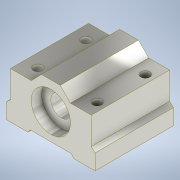
# Autodesk Inventor part: Balero lineal
Saved by Autodesk Inventor 2022 (Build 260153000, 153)
## iProperties
Created: 2021-11-08
Part Number: Balero lineal
Material: Steel
Document SubType Name: Modeling
Designer: Samuel Gómez
Density: 7.85 g/cm^3
Appearance: Silver
Author: Samuel Gómez
Autodesk Inventor part; units mm, degrees
ref_plane "YZ Plane" through (0, 0, 0) normal (1, 0, 0) x (0, 1, 0)
ref_plane "XZ Plane" through (0, 0, 0) normal (0, 1, 0) x (-1, 0, 0)
ref_plane "XY Plane" through (0, 0, 0) normal (0, 0, 1) x (1, 0, 0)
sketch "Boceto1" plane through (0, 0, 0) normal (0, 0, 1) x (1, 0, 0)
  line L0 (0, 0) -> (0, 21.3669) construction
  line L1 (-16.98, 0) -> (-16.98, 6)
  line L2 (-16.98, 0) -> (-8.78, 0)
  line L3 (-16.98, 6) -> (-15.5, 7.35)
  line L4 (-8.78, 0) -> (-7.9, 1.17)
  line L5 (-15.5, 7.35) -> (-15.5, 17.75)
  line L6 (0, 0) -> (-2.9907, 0) construction
  line L7 (-7.9, 1.17) -> (0, 1.17)
  line L8 (-15.5, 17.75) -> (-7.5, 17.75)
  line L9 (-7.5, 17.75) -> (-3.6, 21.72)
  line L10 (-3.6, 21.72) -> (0, 21.72)
  circle A0 centre (0, 11.12) radius 7.5
  line L11 (0, 18.62) -> (5.9047, 18.62) construction
  line L12 (16.98, 0) -> (16.98, 6)
  line L13 (16.98, 0) -> (8.78, 0)
  line L14 (16.98, 6) -> (15.5, 7.35)
  line L15 (8.78, 0) -> (7.9, 1.17)
  line L16 (15.5, 7.35) -> (15.5, 17.75)
  line L17 (7.9, 1.17) -> (0, 1.17)
  line L18 (15.5, 17.75) -> (7.5, 17.75)
  line L19 (7.5, 17.75) -> (3.6, 21.72)
  line L20 (3.6, 21.72) -> (0, 21.72)
  dimension "d12" = 15
  dimension "d0" = 16.98
  dimension "d1" = 6
  dimension "d2" = 15.5
  dimension "d4" = 8.2
  dimension "d6" = 17.75
  dimension "d7" = 10.4
  dimension "d8" = 7.9
  dimension "d9" = 7.5
  dimension "d10" = 21.72
  dimension "d11" = 3.6
  dimension "d13" = 3.1
  dimension "d14" = 20.55
  constraints: 42 end point, 8 symmetric about line, 5 horizontal, 4 point on line, 3 vertical, 1 collinear, 1 perpendicular, 1 vertical alignment, 2 other
  measures "d0" distance between parallel lines of L0 L1
  measures "d1" distance of L1.start L1.end
  measures "d2" distance from line of L0 L3.end
  measures "d4" distance of L1.start L2.end
  measures "d6" vertical distance of L1.start L5.end
  measures "d7" distance of L3.end L5.end
  measures "d8" distance from line of L0 L4.end
  measures "d9" distance from line of L0 L8.end
  measures "d10" distance from line of L1.start L10
  measures "d11" distance of L9.end L10.end
  measures "d13" distance between parallel lines of L11 L10
  measures "d14" distance between parallel lines of L7 L10
extrude "Extrusión1" add sketch "Boceto1" along normal blind 30
sketch "Boceto2" plane through (7.5, 17.75, 0) normal (0, 1, 0) x (1, 0, 0)
  line L0 (1.28, -30) -> (9.48, -30) projected
  line L1 (6.6, -30) -> (6.6, -7.6677) construction
  line L2 (8, 0) -> (8, -30) projected
  line L3 (6.6, -26.3) -> (-1.7379, -26.3) construction
  circle A0 centre (4.85, -24.55) radius 1.75
  line L4 (0.4, 0) -> (0.4, -30) projected
  line L5 (4.85, -22.8) -> (4.85, -7.9) construction
  line L6 (4.85, -7.9) -> (4.85, -6.15) construction
  circle A1 centre (4.85, -6.15) radius 1.75
  line L7 (4.85, -6.15) -> (-16.15, -6.15) construction
  line L8 (-16.15, -6.15) -> (-17.9, -6.15) construction
  circle A2 centre (-17.9, -6.15) radius 1.75
  line L9 (4.85, -24.55) -> (-17.9, -24.55) construction
  line L10 (-17.9, -24.55) -> (-17.9, -6.15) construction
  circle A3 centre (-17.9, -24.55) radius 1.75
  point P0 (-7.5, 0)
  dimension "d19" = 3.5
  dimension "d17" = 1.4
  dimension "d18" = 3.7
  dimension "d20" = 14.9
  dimension "d21" = 1.75
  dimension "d22" = 3.15
  dimension "d23" = 21
  dimension "d24" = 1.75
  dimension "d25" = 3.5
  constraints: 16 end point, 5 horizontal, 3 coincident, 3 vertical, 2 point on line, 2 vertical alignment, 1 centre point, 1 horizontal alignment, 1 parallel, 1 perpendicular, 6 other
  measures "d17" distance between parallel lines of L1 L2
  measures "d18" distance between parallel lines of L0 L3
  measures "d20" distance of L5.start L5.end
  measures "d21" distance of L5.end L6.end
  measures "d22" distance from line of L2 L7.start
  measures "d23" distance of L7.start L7.end
  measures "d24" distance of L7.end L8.end
  measures "d25" diameter of A3
extrude "Extrusión2" cut sketch "Boceto2" against normal up to surface (17.75 mm away)
ref_plane "Plano de trabajo1" through (0, 0, 26) normal (0, 0, 1) x (1, 0, 0)
sketch "Boceto3" plane through (0, 0, 26) normal (0, 0, 1) x (1, 0, 0)
  circle A0 centre (0, 11.12) radius 7.5 projected
  circle A1 centre (0, 11.12) radius 4
  circle A2 centre (0, 11.12) radius 7.5
  point P0 (0, 0)
  dimension "d29" = 8
  constraints: 2 centre point, 2 coincident, 1 concentric
  measures "d29" diameter of A1
extrude "Extrusión3" add sketch "Boceto3" against normal blind 22
